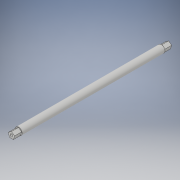
# Autodesk Inventor part: Rod
Saved by Autodesk Inventor 2019.1 (Build 231200000, 200)
## iProperties
Created: 2018-11-25
Part Number: Rod
Material: Generisch
Document SubType Name: Modeling
Designer: JochenAlt
Density: 1 g/cm^3
Appearance: Vorgabe
Author: JochenAlt
Autodesk Inventor part; units mm, degrees
ref_plane "YZ Plane" through (0, 0, 0) normal (1, 0, 0) x (0, 1, 0)
ref_plane "XZ Plane" through (0, 0, 0) normal (0, 1, 0) x (-1, 0, 0)
ref_plane "XY Plane" through (0, 0, 0) normal (0, 0, 1) x (1, 0, 0)
sketch "Skizze1" plane through (0, 0, 0) normal (0, 0, 1) x (1, 0, 0)
  circle A0 centre (0, 0) radius 1.65
  circle A1 centre (0, 0) radius 4.15 construction
  line L0 (0, 4.15) -> (3.9469, 1.2824)
  line L1 (3.9469, 1.2824) -> (2.4393, -3.3574)
  line L2 (2.4393, -3.3574) -> (-2.4393, -3.3574)
  line L3 (-2.4393, -3.3574) -> (-3.9469, 1.2824)
  line L4 (-3.9469, 1.2824) -> (0, 4.15)
  circle A2 centre (0, 0) radius 4.5
  dimension "d1" = 8.3
  dimension "d0" = 3.3
  dimension "d2" = 9
  constraints: 10 end point, 4 coincident, 2 centre point, 1 vertical alignment, 13 other
  measures "d0" diameter of A0
  measures "d2" diameter of A2
extrude "Extrusion1" add sketch "Skizze1" along normal blind 180 contours L0 L1 L2 L3 L4 | A2
extrude "Extrusion2" add sketch "Skizze1" against normal blind 9 contours L0 L1 L2 L3 L4
extrude "Extrusion3" add sketch "Skizze1" along normal blind 9 from surface at 180 contours L0 L1 L2 L3 L4
